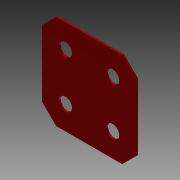
# Autodesk Inventor part: Preview Plate
Saved by Autodesk Inventor 2013 (Build 170138000, 138)
## iProperties
Created: 2013-04-04
Part Number: Preview Plate
Material: Generic
Document SubType Name: Modeling
Designer: mvarma
Density: 1 g/cm^3
Author: mvarma
Autodesk Inventor part; units mm, degrees
ref_plane "YZ Plane" through (0, 0, 0) normal (1, 0, 0) x (0, 1, 0)
ref_plane "XZ Plane" through (0, 0, 0) normal (0, 1, 0) x (-1, 0, 0)
ref_plane "XY Plane" through (0, 0, 0) normal (0, 0, 1) x (1, 0, 0)
sketch "Sketch1" plane through (0, 0, 0) normal (0, 0, 1) x (1, 0, 0)
  line L0 (0, 0) -> (254, 0)
  line L1 (254, 0) -> (254, -254)
  line L2 (254, -254) -> (0, -254)
  line L3 (0, -254) -> (0, 0)
  circle A0 centre (63.5, -63.5) radius 17.4625
  circle A1 centre (190.5, -63.5) radius 17.4625
  circle A2 centre (63.5, -190.5) radius 17.4625
  circle A3 centre (190.5, -190.5) radius 17.4625
  line L4 (127, 0) -> (127, -254) construction
  line L5 (0, -127) -> (254, -127) construction
  line L6 (190.5, 0) -> (190.5, -254) construction
  line L7 (63.5, 0) -> (63.5, -254) construction
  line L8 (0, -190.5) -> (254, -190.5) construction
  line L9 (0, -63.5) -> (254, -63.5) construction
  dimension "d0" = 254
  dimension "d1" = 254
  dimension "d2" = 34.925
  dimension "d3" = 34.925
  dimension "d4" = 34.925
  dimension "d5" = 34.925
  dimension "d6" = 63.5
  dimension "d7" = 63.5
  dimension "d9" = 63.5
  dimension "d10" = 63.5
  constraints: 20 end point, 16 point on line, 5 perpendicular, 4 centre point, 4 midpoint, 2 parallel, 1 horizontal
  measures "d0" distance of L0.end L1.end
  measures "d1" distance of L1.end L2.end
  measures "d2" diameter of A2
  measures "d3" diameter of A0
  measures "d4" diameter of A1
  measures "d5" diameter of A3
  measures "d6" distance between parallel lines of L0 L9
  measures "d7" distance between parallel lines of L1 L6
  measures "d9" distance between parallel lines of L2 L8
  measures "d10" distance between parallel lines of L3 L7
extrude "Extrusion1" add sketch "Sketch1" along normal blind 4.7625
chamfer "Chamfer1" distance 38.1 angle 45 4 edges at (0, 0, 2.3813) (0, -254, 2.3813) (254, -254, 2.3813) (254, 0, 2.3813)
equation "\"d7\" = d6"
equation "\"d9\" = d8"
equation "\"d10\" = d9"
equation "\"d8\" = d7"
body "Solid1"
